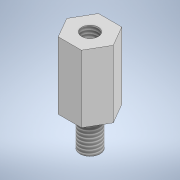
# Autodesk Inventor part: Spacer10mm
Saved by Autodesk Inventor 2022 (Build 260153000, 153)
## iProperties
Created: 2022-04-20
Part Number: Spacer10mm
Material: Generic
Document SubType Name: Modeling
Designer: Yazawa
Density: 1 g/cm^3
Appearance: Default
Author: Yazawa
Autodesk Inventor part; units mm, degrees
ref_plane "YZ Plane" through (0, 0, 0) normal (1, 0, 0) x (0, 1, 0)
ref_plane "XZ Plane" through (0, 0, 0) normal (0, 1, 0) x (-1, 0, 0)
ref_plane "XY Plane" through (0, 0, 0) normal (0, 0, 1) x (1, 0, 0)
sketch "スケッチ1" plane through (0, 0, 0) normal (0, 1, 0) x (-1, 0, 0)
  line L0 (1.7321, -3) -> (-1.7321, -3)
  line L1 (-1.7321, -3) -> (-3.4641, 0)
  line L2 (-3.4641, 0) -> (-1.7321, 3)
  line L3 (-1.7321, 3) -> (1.7321, 3)
  line L4 (1.7321, 3) -> (3.4641, 0)
  line L5 (3.4641, 0) -> (1.7321, -3)
  line L6 (1.7321, -3) -> (-1.7321, 3) construction
  line L7 (-3.4641, 0) -> (3.4641, 0) construction
  line L8 (-1.7321, -3) -> (1.7321, 3) construction
  point P0 (0, 0)
  point P1 (0, 0)
  point P2 (0, 0)
  dimension "d0" = 6
  constraints: 18 end point, 7 equal length, 3 midpoint, 1 coincident, 1 horizontal, 1 parallel
  measures "d0" distance between parallel lines of L3 L0
extrude "押し出し1" add sketch "スケッチ1" along normal blind 10
sketch "スケッチ2" plane through (0, 10, 0) normal (0, 1, 0) x (1, 0, 0)
  point P0 (0, 0)
  point P1 (0, 0)
  constraints: 1 coincident
hole "穴1" at (0, 10, 0) direction (0, -1, 0) diameter 2.459 depth 4.8 thread size "M3x0.5" class "6H" standard "ISO Metric profile"
sketch "スケッチ3" plane through (0, 0, 0) normal (0, -1, 0) x (1, 0, 0)
  circle A0 centre (0, 0) radius 1.5
  dimension "d10" = 3
  constraints: 1 centre point, 1 coincident
  measures "d10" diameter of A0
extrude "押し出し2" add sketch "スケッチ3" along normal blind 5
thread "ねじ1" size "M3x0.5" class "6g" standard "ISO Metric profile" full length
